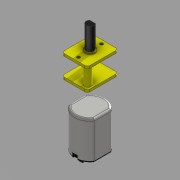
# Autodesk Inventor part: Pololu Metal Gearmotor
Saved by Autodesk Inventor 2013 SP2 (Build 170200200, 200)
## iProperties
Created: 2014-04-15
Part Number: Pololu Metal Gearmotor
Material: Generic
Document SubType Name: Modeling
Designer: Kevin
Density: 1 g/cm^3
Author: Kevin
Autodesk Inventor part; units mm, degrees
ref_plane "YZ Plane" through (0, 0, 0) normal (1, 0, 0) x (0, 1, 0)
ref_plane "XZ Plane" through (0, 0, 0) normal (0, 1, 0) x (-1, 0, 0)
ref_plane "XY Plane" through (0, 0, 0) normal (0, 0, 1) x (1, 0, 0)
sketch "Sketch1" plane through (0, 0, 0) normal (0, 0, 1) x (1, 0, 0)
  line L0 (1, 0) -> (9, 0)
  line L1 (10, 1) -> (10, 11)
  line L2 (9, 12) -> (1, 12)
  line L3 (0, 11) -> (0, 1)
  arc A0 (10, 11) -> (9, 12) centre (9, 11) ccw
  arc A1 (1, 12) -> (0, 11) centre (1, 11) ccw
  arc A2 (9, 0) -> (10, 1) centre (9, 1) ccw
  arc A3 (0, 1) -> (1, 0) centre (1, 1) ccw
  point P0 (0, 0)
  point P1 (10, 12)
  point P2 (10, 0)
  point P3 (0, 12)
  dimension "d0" = 10
  dimension "d1" = 12
  dimension "d2" = 1
  dimension "d3" = 1
  constraints: 8 end point, 8 point on circle, 8 point on line, 8 tangent, 4 centre point, 2 equal radius, 2 parallel, 1 horizontal, 1 perpendicular
  measures "d0" distance of point (0, 12) point (10, 12)
  measures "d1" distance of point (10, 12) point (10, 0)
  measures "d2" radius of A0
  measures "d3" radius of A3
extrude "Extrusion1" add sketch "Sketch1" against normal blind 1
sketch "Sketch2" plane through (0, 0, -1) normal (0, 0, -1) x (-1, 0, 0)
  line L0 (-10, 11) -> (-10, 1) projected
  line L1 (-9, 0) -> (-1, 0) projected
  line L2 (0, 1) -> (0, 11) projected
  line L3 (-1, 12) -> (-9, 12) projected
  line L4 (0.1733, 12) -> (-1.8267, 12)
  line L5 (-1.8267, 12) -> (-1.8267, 10)
  circle A0 centre (-1.8267, 10) radius 1.25
  line L6 (0, 6) -> (-10, 6)
  line L7 (-5, 12) -> (-5, 0)
  circle A1 centre (-8.1733, 2) radius 1.25
  point P0 (0, 0)
  point P1 (-5, 6)
  point P2 (-5, 6)
  dimension "d6" = 2
  dimension "d7" = 2
  dimension "d8" = 2.5
  dimension "d11" = 360
  constraints: 8 end point, 5 midpoint, 2 centre point, 2 coincident, 1 perpendicular, 1 point on line, 5 other
  measures "d6" distance of L4.start L4.end
  measures "d7" distance of L4.end L5.end
  measures "d8" diameter of A0
extrude "Extrusion2" add sketch "Sketch2" along normal blind 7
sketch "Sketch3" plane through (1.8267, 10, -8) normal (0, 0, -1) x (-1, 0, 0)
  line L0 (0.8267, -10) -> (-7.1733, -10)
  line L1 (-8.1733, -9) -> (-8.1733, 1)
  line L2 (-7.1733, 2) -> (0.8267, 2)
  line L3 (1.8267, 1) -> (1.8267, -9)
  arc A0 (-7.1733, 2) -> (-8.1733, 1) centre (-7.1733, 1) ccw
  arc A1 (1.8267, 1) -> (0.8267, 2) centre (0.8267, 1) ccw
  arc A2 (-8.1733, -9) -> (-7.1733, -10) centre (-7.1733, -9) ccw
  arc A3 (0.8267, -10) -> (1.8267, -9) centre (0.8267, -9) ccw
  point P0 (1.8267, -10)
  point P1 (-8.1733, 2)
  point P2 (-8.1733, -10)
  point P3 (1.8267, 2)
  dimension "d15" = 10
  dimension "d16" = 12
  dimension "d17" = 1
  constraints: 8 end point, 8 point on circle, 8 point on line, 8 tangent, 4 centre point, 3 equal radius, 2 parallel, 1 horizontal, 1 perpendicular
  measures "d15" distance of point (-8.173, 2) point (1.827, 2)
  measures "d16" distance of point (-8.173, -10) point (-8.173, 2)
  measures "d17" radius of A0
extrude "Extrusion3" add sketch "Sketch3" along normal blind 1
sketch "Sketch4" plane through (0, 0, 0) normal (0, 0, 1) x (1, 0, 0)
  line L0 (10, 11) -> (10, 1) projected
  line L1 (0, 1) -> (0, 11) projected
  line L2 (0, 6) -> (10, 6)
  circle A0 centre (5, 6) radius 1.95
  point P0 (0, 0)
  dimension "d20" = 3.9
  constraints: 3 midpoint, 2 end point, 1 centre point
  measures "d20" diameter of A0
extrude "Extrusion4" add sketch "Sketch4" along normal blind 0.6
chamfer "Chamfer1" distance 0.2 angle 45 1 edges at (3.05, 6, 0.6)
sketch "Sketch5" plane through (5, 6, 0.6) normal (0, 0, 1) x (1, 0, 0)
  circle A0 centre (0, 0) radius 1.75 projected
  circle A1 centre (0, 0) radius 1.5
  line L0 (0, -1.5) -> (0, 1)
  line L1 (-1.118, 1) -> (0, 1)
  line L2 (0, 1) -> (1.118, 1)
  point P0 (-5, -6)
  dimension "d26" = 3
  dimension "d27" = 2.5
  constraints: 6 end point, 3 point on circle, 1 centre point, 1 coincident, 1 collinear, 1 perpendicular, 1 vertical
  measures "d26" diameter of A1
  measures "d27" distance of L0.start L0.end
extrude "Extrusion5" add sketch "Sketch5" along normal blind 8.67 contours A1 L0 L2 | A1 L1 L0
sketch "Sketch6" plane through (0, 0, 0) normal (0, 0, 1) x (1, 0, 0)
  circle A0 centre (5, 6) radius 1.95 projected
  line L0 (9, 0) -> (1, 0) projected
  line L1 (5, 6) -> (5, 10.5)
  point P0 (0, 0)
  dimension "d30" = 4.5
  constraints: 2 end point, 1 perpendicular
  measures "d30" distance of L1.start L1.end
hole "Hole1" at (5, 10.5, 0) direction (0, 0, -1) diameter 1.221 end up to face face through (3.0146, 4.1133, -1) facing (0, 0, -1) thread size "M1.6x0.35" class "6H" standard "ANSI Metric M Profile"
sketch "Sketch8" plane through (0, 0, 0) normal (0, 0, 1) x (1, 0, 0)
  circle A0 centre (5, 6) radius 1.95 projected
  line L0 (9, 0) -> (1, 0) projected
  line L1 (5, 6) -> (5, 1.5)
  point P0 (0, 0)
  dimension "d39" = 4.5
  constraints: 2 end point, 1 perpendicular
  measures "d39" distance of L1.start L1.end
hole "Hole2" at (5, 1.5, 0) direction (0, 0, -1) diameter 1.221 end up to face face through (3.0146, 4.1133, -1) facing (0, 0, -1) thread size "M1.6x0.35" class "6H" standard "ANSI Metric M Profile"
sketch "Sketch9" plane through (1.8267, 10, -9) normal (0, 0, -1) x (-1, 0, 0)
  line L0 (-8.1733, 1) -> (-8.1733, -9) projected
  line L1 (-7.1733, -10) -> (0.8267, -10) projected
  line L2 (1.8267, -9) -> (1.8267, 1) projected
  line L3 (0.8267, 2) -> (-7.1733, 2) projected
  line L4 (-3.1733, 2) -> (-3.1733, -10)
  circle A0 centre (-3.1733, -4) radius 6
  line L5 (-8.1733, -0.6834) -> (-8.1733, -7.3166)
  line L6 (1.8267, -0.6834) -> (1.8267, -7.3166)
  point P0 (1.8267, -10)
  dimension "d47" = 12
  constraints: 6 end point, 4 point on circle, 4 point on line, 3 midpoint, 1 centre point
  measures "d47" diameter of A0
extrude "Extrusion6" add sketch "Sketch9" along normal blind 15 separate body contours A0 L4 L0 | A0 L2 L4
move or copy body "Move Body1" bodies to move or copy 2 copy no translate (0, 0, -10)
fillet "Fillet1" radius 0.75 8 edges at (5, 12, -19) (10, 6, -19) (5, 0, -19) (0, 6, -19) (0, 6, -34) (5, 12, -34) (10, 6, -34) (5, 0, -34)
sketch "Sketch10" plane through (5, 6, -34) normal (0, 0, -1) x (-1, 0, 0)
  arc A0 (4.25, 3.0822) -> (-4.25, 3.0822) centre (0, 0) ccw projected
  circle A1 centre (0, 0) radius 2.5
  point P0 (5, -6)
  dimension "d54" = 5
  constraints: 1 centre point, 1 coincident
  measures "d54" diameter of A1
extrude "Extrusion7" add sketch "Sketch10" along normal blind 2 bodies 2
fillet "Fillet2" radius 1 1 edges at (7.5, 6, -36)
sketch "Sketch11" plane through (5, 6, -36) normal (0, 0, -1) x (-1, 0, 0)
  circle A0 centre (0, 0) radius 1.5 projected
  circle A1 centre (0, 0) radius 1
  point P0 (5, -6)
  dimension "d58" = 2
  constraints: 1 centre point, 1 coincident
  measures "d58" diameter of A1
extrude "Extrusion8" cut sketch "Sketch11" against normal blind 0.5 draft 0.5 contours A1 bodies 2
sketch "Sketch13" plane through (5, 6, -35.5) normal (0, 0, -1) x (-1, 0, 0)
  circle A0 centre (0, 0) radius 1.0044 projected
  circle A1 centre (0, 0) radius 0.5
  point P0 (5, -6)
  dimension "d61" = 1
  constraints: 1 centre point, 1 coincident
  measures "d61" diameter of A1
extrude "Extrusion9" add sketch "Sketch13" along normal blind 0.5 contours A1 bodies 2
sketch "Sketch14" plane through (5, 6, -34) normal (0, 0, -1) x (-1, 0, 0)
  line L0 (4.25, 3.0822) -> (4.25, -3.0822) projected
  arc A0 (4.25, 3.0822) -> (-4.25, 3.0822) centre (0, 0) ccw projected
  line L1 (0, 0) -> (0, 3.5)
  line L2 (0, 3.5) -> (1, 3.5)
  line L3 (1, 3.5) -> (1, 3.6)
  line L4 (1, 3.6) -> (0, 3.6)
  line L5 (0, 3.6) -> (0, 3.5)
  line L6 (0, 3.5) -> (-1, 3.5)
  line L7 (-1, 3.5) -> (-1, 3.6)
  line L8 (-1, 3.6) -> (0, 3.6)
  line L9 (0, 3.6) -> (0, 3.5)
  point P0 (5, -6)
  dimension "d64" = 3.5
  dimension "d65" = 1
  dimension "d66" = 0.1
  dimension "d67" = 1
  dimension "d68" = 0.1
  constraints: 18 end point, 5 parallel, 2 horizontal, 2 perpendicular
  measures "d64" distance of L1.start L1.end
  measures "d65" distance of L4.end L3.end
  measures "d66" distance of L3.end L2.end
  measures "d67" distance of L7.end L8.end
  measures "d68" distance of L6.end L7.end
extrude "Extrusion10" add sketch "Sketch14" along normal blind 2 bodies 2
sketch "Sketch15" plane through (4, 9.6, -34) normal (0, 1, 0) x (1, 0, 0)
  circle A0 centre (1, 1) radius 0.625
  point P0 (-4, -34)
  dimension "d71" = 1.25
  constraints: 1 centre point
  measures "d71" diameter of A0
extrude "Extrusion11" cut sketch "Sketch15" against normal blind 0.1 bodies 2
fillet "Fillet3" radius 0.5 2 edges at (4, 9.55, -36) (6, 9.55, -36)
sketch "Sketch16" plane through (5, 6, -34) normal (0, 0, -1) x (-1, 0, 0)
  line L0 (4.25, 3.0822) -> (4.25, -3.0822) projected
  arc A0 (4.25, 3.0822) -> (-4.25, 3.0822) centre (0, 0) ccw projected
  line L1 (0, 0) -> (0, 6)
  line L2 (0, 6) -> (1, 6)
  line L3 (1, 6) -> (1, 5)
  line L4 (1, 5) -> (0, 5)
  line L5 (0, 5) -> (0, 6)
  line L6 (0, 6) -> (-1, 6)
  line L7 (-1, 6) -> (-1, 5)
  line L8 (-1, 5) -> (0, 5)
  line L9 (0, 5) -> (0, 6)
  point P0 (5, -6)
  dimension "d75" = 6
  dimension "d76" = 1
  dimension "d77" = 1
  dimension "d78" = 1
  dimension "d79" = 1
  constraints: 18 end point, 5 parallel, 2 horizontal, 2 perpendicular
  measures "d75" distance of L1.start L1.end
  measures "d76" distance of L3.end L4.end
  measures "d77" distance of L2.end L3.end
  measures "d78" distance of L8.end L7.end
  measures "d79" distance of L7.end L6.end
extrude "Extrusion12" cut sketch "Sketch16" against normal blind 2 bodies 2
pattern_circular "Circular Pattern1" count 2 over 360 about axis through (5, 6, -35.5) along (0, 0, -1) of "Extrusion10", "Extrusion11", "Fillet3", "Extrusion12" bodies 2
body "Solid1"
body "Solid2"
